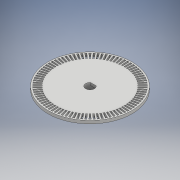
# Autodesk Inventor part: Ответная часть энкодера(колесо)
Saved by Autodesk Inventor 2018 (Build 220112000, 112)
## iProperties
Created: 2018-12-06
Part Number: Ответная часть энкодера(колесо)
Material: Типовые
Document SubType Name: Modeling
Designer: RR
Density: 1 g/cm^3
Appearance: По умолчанию
Author: RR
Autodesk Inventor part; units mm, degrees
ref_plane "YZ Plane" through (0, 0, 0) normal (1, 0, 0) x (0, 1, 0)
ref_plane "XZ Plane" through (0, 0, 0) normal (0, 1, 0) x (-1, 0, 0)
ref_plane "XY Plane" through (0, 0, 0) normal (0, 0, 1) x (1, 0, 0)
sketch "Эскиз1" plane through (0, 0, 0) normal (0, 0, 1) x (1, 0, 0)
  circle A0 centre (0, 0) radius 28
  arc A1 (1, 27.4818) -> (0, 27.5) centre (0, 0) ccw
  line L0 (0, 27.5) -> (1, 27.4818)
  arc A2 (0.8364, 22.9848) -> (0, 23) centre (0, 0) ccw
  line L1 (0, 2.3) -> (1.9261, 2.3) construction
  line L2 (1, 27.4818) -> (0.8364, 22.9848)
  line L3 (0, 23) -> (0, 27.5)
  arc A3 (-1.0087, 27.4815) -> (-2.0074, 27.4266) centre (0, 0) ccw
  line L4 (-2.0074, 27.4266) -> (-1.0087, 27.4815)
  arc A4 (-0.8436, 22.9845) -> (-1.6789, 22.9386) centre (0, 0) ccw
  line L5 (-1.0087, 27.4815) -> (-0.8436, 22.9845)
  line L6 (-1.6789, 22.9386) -> (-2.0074, 27.4266)
  arc A5 (-3.012, 27.3345) -> (-4.004, 27.2069) centre (0, 0) ccw
  line L7 (-4.004, 27.2069) -> (-3.012, 27.3345)
  arc A6 (-2.5192, 22.8616) -> (-3.3488, 22.7549) centre (0, 0) ccw
  line L8 (-3.012, 27.3345) -> (-2.5192, 22.8616)
  line L9 (-3.3488, 22.7549) -> (-4.004, 27.2069)
  arc A7 (-4.9993, 27.0418) -> (-5.9793, 26.8421) centre (0, 0) ccw
  line L10 (-5.9793, 26.8421) -> (-4.9993, 27.0418)
  arc A8 (-4.1812, 22.6167) -> (-5.0009, 22.4497) centre (0, 0) ccw
  line L11 (-4.9993, 27.0418) -> (-4.1812, 22.6167)
  line L12 (-5.0009, 22.4497) -> (-5.9793, 26.8421)
  arc A9 (-6.9599, 26.6047) -> (-7.9227, 26.334) centre (0, 0) ccw
  line L13 (-7.9227, 26.334) -> (-6.9599, 26.6047)
  arc A10 (-5.821, 22.2512) -> (-6.6263, 22.0248) centre (0, 0) ccw
  line L14 (-6.9599, 26.6047) -> (-5.821, 22.2512)
  line L15 (-6.6263, 22.0248) -> (-7.9227, 26.334)
  arc A11 (-8.8833, 26.0257) -> (-9.8238, 25.6854) centre (0, 0) ccw
  line L16 (-9.8238, 25.6854) -> (-8.8833, 26.0257)
  arc A12 (-7.4297, 21.7669) -> (-8.2163, 21.4824) centre (0, 0) ccw
  line L17 (-8.8833, 26.0257) -> (-7.4297, 21.7669)
  line L18 (-8.2163, 21.4824) -> (-9.8238, 25.6854)
  arc A13 (-10.7594, 25.3078) -> (-11.6726, 24.8998) centre (0, 0) ccw
  line L19 (-11.6726, 24.8998) -> (-10.7594, 25.3078)
  arc A14 (-8.9988, 21.1665) -> (-9.7625, 20.8253) centre (0, 0) ccw
  line L20 (-10.7594, 25.3078) -> (-8.9988, 21.1665)
  line L21 (-9.7625, 20.8253) -> (-11.6726, 24.8998)
  arc A15 (-12.578, 24.4549) -> (-13.459, 23.9814) centre (0, 0) ccw
  line L22 (-13.459, 23.9814) -> (-12.578, 24.4549)
  arc A16 (-10.5198, 20.4532) -> (-11.2566, 20.0571) centre (0, 0) ccw
  line L23 (-12.578, 24.4549) -> (-10.5198, 20.4532)
  line L24 (-11.2566, 20.0571) -> (-13.459, 23.9814)
  arc A17 (-14.3296, 23.4715) -> (-15.1736, 22.9349) centre (0, 0) ccw
  line L25 (-15.1736, 22.9349) -> (-14.3296, 23.4715)
  arc A18 (-11.9847, 19.6307) -> (-12.6907, 19.1819) centre (0, 0) ccw
  line L26 (-14.3296, 23.4715) -> (-11.9847, 19.6307)
  line L27 (-12.6907, 19.1819) -> (-15.1736, 22.9349)
  arc A19 (-16.0047, 22.3629) -> (-16.8073, 21.7662) centre (0, 0) ccw
  line L28 (-16.8073, 21.7662) -> (-16.0047, 22.3629)
  arc A20 (-13.3857, 18.7035) -> (-14.057, 18.2044) centre (0, 0) ccw
  line L29 (-16.0047, 22.3629) -> (-13.3857, 18.7035)
  line L30 (-14.057, 18.2044) -> (-16.8073, 21.7662)
  arc A21 (-17.5944, 21.135) -> (-18.3513, 20.4812) centre (0, 0) ccw
  line L31 (-18.3513, 20.4812) -> (-17.5944, 21.135)
  arc A22 (-14.7153, 17.6766) -> (-15.3483, 17.1298) centre (0, 0) ccw
  line L32 (-17.5944, 21.135) -> (-14.7153, 17.6766)
  line L33 (-15.3483, 17.1298) -> (-18.3513, 20.4812)
  arc A23 (-19.0902, 19.7943) -> (-19.7973, 19.087) centre (0, 0) ccw
  line L34 (-19.7973, 19.087) -> (-19.0902, 19.7943)
  arc A24 (-15.9663, 16.5552) -> (-16.5578, 15.9637) centre (0, 0) ccw
  line L35 (-19.0902, 19.7943) -> (-15.9663, 16.5552)
  line L36 (-16.5578, 15.9637) -> (-19.7973, 19.087)
  arc A25 (-20.4841, 18.348) -> (-21.1378, 17.591) centre (0, 0) ccw
  line L37 (-21.1378, 17.591) -> (-20.4841, 18.348)
  arc A26 (-17.1322, 15.3456) -> (-17.6789, 14.7125) centre (0, 0) ccw
  line L38 (-20.4841, 18.348) -> (-17.1322, 15.3456)
  line L39 (-17.6789, 14.7125) -> (-21.1378, 17.591)
  arc A27 (-21.7688, 16.8038) -> (-22.3655, 16.0011) centre (0, 0) ccw
  line L40 (-22.3655, 16.0011) -> (-21.7688, 16.8038)
  arc A28 (-18.2066, 14.0541) -> (-18.7057, 13.3828) centre (0, 0) ccw
  line L41 (-21.7688, 16.8038) -> (-18.2066, 14.0541)
  line L42 (-18.7057, 13.3828) -> (-22.3655, 16.0011)
  arc A29 (-22.9373, 15.17) -> (-23.4738, 14.3259) centre (0, 0) ccw
  line L43 (-23.4738, 14.3259) -> (-22.9373, 15.17)
  arc A30 (-19.184, 12.6876) -> (-19.6326, 11.9816) centre (0, 0) ccw
  line L44 (-22.9373, 15.17) -> (-19.184, 12.6876)
  line L45 (-19.6326, 11.9816) -> (-23.4738, 14.3259)
  arc A31 (-23.9835, 13.4552) -> (-24.4569, 12.5742) centre (0, 0) ccw
  line L46 (-24.4569, 12.5742) -> (-23.9835, 13.4552)
  arc A32 (-20.0589, 11.2534) -> (-20.4549, 10.5166) centre (0, 0) ccw
  line L47 (-23.9835, 13.4552) -> (-20.0589, 11.2534)
  line L48 (-20.4549, 10.5166) -> (-24.4569, 12.5742)
  arc A33 (-24.9017, 11.6686) -> (-25.3095, 10.7554) centre (0, 0) ccw
  line L49 (-25.3095, 10.7554) -> (-24.9017, 11.6686)
  arc A34 (-20.8269, 9.7592) -> (-21.168, 8.9954) centre (0, 0) ccw
  line L50 (-24.9017, 11.6686) -> (-20.8269, 9.7592)
  line L51 (-21.168, 8.9954) -> (-25.3095, 10.7554)
  arc A35 (-25.687, 9.8198) -> (-26.0271, 8.8792) centre (0, 0) ccw
  line L52 (-26.0271, 8.8792) -> (-25.687, 9.8198)
  arc A36 (-21.4837, 8.2129) -> (-21.7681, 7.4262) centre (0, 0) ccw
  line L53 (-25.687, 9.8198) -> (-21.4837, 8.2129)
  line L54 (-21.7681, 7.4262) -> (-26.0271, 8.8792)
  arc A37 (-26.3353, 7.9186) -> (-26.6058, 6.9557) centre (0, 0) ccw
  line L55 (-26.6058, 6.9557) -> (-26.3353, 7.9186)
  arc A38 (-22.0259, 6.6228) -> (-22.2521, 5.8175) centre (0, 0) ccw
  line L56 (-26.3353, 7.9186) -> (-22.0259, 6.6228)
  line L57 (-22.2521, 5.8175) -> (-26.6058, 6.9557)
  arc A39 (-26.843, 5.9751) -> (-27.0426, 4.995) centre (0, 0) ccw
  line L58 (-27.0426, 4.995) -> (-26.843, 5.9751)
  arc A40 (-22.4505, 4.9973) -> (-22.6174, 4.1776) centre (0, 0) ccw
  line L59 (-26.843, 5.9751) -> (-22.4505, 4.9973)
  line L60 (-22.6174, 4.1776) -> (-27.0426, 4.995)
  arc A41 (-27.2076, 3.9997) -> (-27.335, 3.0077) centre (0, 0) ccw
  line L61 (-27.335, 3.0077) -> (-27.2076, 3.9997)
  arc A42 (-22.7554, 3.3452) -> (-22.862, 2.5155) centre (0, 0) ccw
  line L62 (-27.2076, 3.9997) -> (-22.7554, 3.3452)
  line L63 (-22.862, 2.5155) -> (-27.335, 3.0077)
  arc A43 (-27.427, 2.003) -> (-27.4817, 1.0044) centre (0, 0) ccw
  line L64 (-27.4817, 1.0044) -> (-27.427, 2.003)
  arc A44 (-22.9389, 1.6753) -> (-22.9847, 0.84) centre (0, 0) ccw
  line L65 (-27.427, 2.003) -> (-22.9389, 1.6753)
  line L66 (-22.9847, 0.84) -> (-27.4817, 1.0044)
  arc A45 (-27.5, -0.0044) -> (-27.4817, -1.0044) centre (0, 0) ccw
  line L67 (-27.4817, -1.0044) -> (-27.5, -0.0044)
  arc A46 (-23, -0.0036) -> (-22.9847, -0.84) centre (0, 0) ccw
  line L68 (-27.5, -0.0044) -> (-23, -0.0036)
  line L69 (-22.9847, -0.84) -> (-27.4817, -1.0044)
  arc A47 (-27.4263, -2.0117) -> (-27.335, -3.0077) centre (0, 0) ccw
  line L70 (-27.335, -3.0077) -> (-27.4263, -2.0117)
  arc A48 (-22.9384, -1.6825) -> (-22.862, -2.5155) centre (0, 0) ccw
  line L71 (-27.4263, -2.0117) -> (-22.9384, -1.6825)
  line L72 (-22.862, -2.5155) -> (-27.335, -3.0077)
  arc A49 (-27.2063, -4.0083) -> (-27.0426, -4.995) centre (0, 0) ccw
  line L73 (-27.0426, -4.995) -> (-27.2063, -4.0083)
  arc A50 (-22.7544, -3.3524) -> (-22.6174, -4.1776) centre (0, 0) ccw
  line L74 (-27.2063, -4.0083) -> (-22.7544, -3.3524)
  line L75 (-22.6174, -4.1776) -> (-27.0426, -4.995)
  arc A51 (-26.8411, -5.9836) -> (-26.6058, -6.9557) centre (0, 0) ccw
  line L76 (-26.6058, -6.9557) -> (-26.8411, -5.9836)
  arc A52 (-22.449, -5.0045) -> (-22.2521, -5.8175) centre (0, 0) ccw
  line L77 (-26.8411, -5.9836) -> (-22.449, -5.0045)
  line L78 (-22.2521, -5.8175) -> (-26.6058, -6.9557)
  arc A53 (-26.3328, -7.9269) -> (-26.0271, -8.8792) centre (0, 0) ccw
  line L79 (-26.0271, -8.8792) -> (-26.3328, -7.9269)
  arc A54 (-22.0238, -6.6298) -> (-21.7681, -7.4262) centre (0, 0) ccw
  line L80 (-26.3328, -7.9269) -> (-22.0238, -6.6298)
  line L81 (-21.7681, -7.4262) -> (-26.0271, -8.8792)
  arc A55 (-25.6839, -9.8279) -> (-25.3095, -10.7554) centre (0, 0) ccw
  line L82 (-25.3095, -10.7554) -> (-25.6839, -9.8279)
  arc A56 (-21.4811, -8.2197) -> (-21.168, -8.9954) centre (0, 0) ccw
  line L83 (-25.6839, -9.8279) -> (-21.4811, -8.2197)
  line L84 (-21.168, -8.9954) -> (-25.3095, -10.7554)
  arc A57 (-24.898, -11.6765) -> (-24.4569, -12.5742) centre (0, 0) ccw
  line L85 (-24.4569, -12.5742) -> (-24.898, -11.6765)
  arc A58 (-20.8238, -9.7658) -> (-20.4549, -10.5166) centre (0, 0) ccw
  line L86 (-24.898, -11.6765) -> (-20.8238, -9.7658)
  line L87 (-20.4549, -10.5166) -> (-24.4569, -12.5742)
  arc A59 (-23.9792, -13.4628) -> (-23.4738, -14.3259) centre (0, 0) ccw
  line L88 (-23.4738, -14.3259) -> (-23.9792, -13.4628)
  arc A60 (-20.0554, -11.2598) -> (-19.6326, -11.9816) centre (0, 0) ccw
  line L89 (-23.9792, -13.4628) -> (-20.0554, -11.2598)
  line L90 (-19.6326, -11.9816) -> (-23.4738, -14.3259)
  arc A61 (-22.9325, -15.1772) -> (-22.3655, -16.0011) centre (0, 0) ccw
  line L91 (-22.3655, -16.0011) -> (-22.9325, -15.1772)
  arc A62 (-19.1799, -12.6937) -> (-18.7057, -13.3828) centre (0, 0) ccw
  line L92 (-22.9325, -15.1772) -> (-19.1799, -12.6937)
  line L93 (-18.7057, -13.3828) -> (-22.3655, -16.0011)
  arc A63 (-21.7635, -16.8107) -> (-21.1378, -17.591) centre (0, 0) ccw
  line L94 (-21.1378, -17.591) -> (-21.7635, -16.8107)
  arc A64 (-18.2022, -14.0599) -> (-17.6789, -14.7125) centre (0, 0) ccw
  line L95 (-21.7635, -16.8107) -> (-18.2022, -14.0599)
  line L96 (-17.6789, -14.7125) -> (-21.1378, -17.591)
  arc A65 (-20.4783, -18.3545) -> (-19.7973, -19.087) centre (0, 0) ccw
  line L97 (-19.7973, -19.087) -> (-20.4783, -18.3545)
  arc A66 (-17.1273, -15.351) -> (-16.5578, -15.9637) centre (0, 0) ccw
  line L98 (-20.4783, -18.3545) -> (-17.1273, -15.351)
  line L99 (-16.5578, -15.9637) -> (-19.7973, -19.087)
  arc A67 (-19.0839, -19.8004) -> (-18.3513, -20.4812) centre (0, 0) ccw
  line L100 (-18.3513, -20.4812) -> (-19.0839, -19.8004)
  arc A68 (-15.9611, -16.5603) -> (-15.3483, -17.1298) centre (0, 0) ccw
  line L101 (-19.0839, -19.8004) -> (-15.9611, -16.5603)
  line L102 (-15.3483, -17.1298) -> (-18.3513, -20.4812)
  arc A69 (-17.5877, -21.1406) -> (-16.8073, -21.7662) centre (0, 0) ccw
  line L103 (-16.8073, -21.7662) -> (-17.5877, -21.1406)
  arc A70 (-14.7097, -17.6812) -> (-14.057, -18.2044) centre (0, 0) ccw
  line L104 (-17.5877, -21.1406) -> (-14.7097, -17.6812)
  line L105 (-14.057, -18.2044) -> (-16.8073, -21.7662)
  arc A71 (-15.9976, -22.368) -> (-15.1736, -22.9349) centre (0, 0) ccw
  line L106 (-15.1736, -22.9349) -> (-15.9976, -22.368)
  arc A72 (-13.3798, -18.7078) -> (-12.6907, -19.1819) centre (0, 0) ccw
  line L107 (-15.9976, -22.368) -> (-13.3798, -18.7078)
  line L108 (-12.6907, -19.1819) -> (-15.1736, -22.9349)
  arc A73 (-14.3221, -23.4761) -> (-13.459, -23.9814) centre (0, 0) ccw
  line L109 (-13.459, -23.9814) -> (-14.3221, -23.4761)
  arc A74 (-11.9785, -19.6345) -> (-11.2566, -20.0571) centre (0, 0) ccw
  line L110 (-14.3221, -23.4761) -> (-11.9785, -19.6345)
  line L111 (-11.2566, -20.0571) -> (-13.459, -23.9814)
  arc A75 (-12.5703, -24.4589) -> (-11.6726, -24.8998) centre (0, 0) ccw
  line L112 (-11.6726, -24.8998) -> (-12.5703, -24.4589)
  arc A76 (-10.5133, -20.4565) -> (-9.7625, -20.8253) centre (0, 0) ccw
  line L113 (-12.5703, -24.4589) -> (-10.5133, -20.4565)
  line L114 (-9.7625, -20.8253) -> (-11.6726, -24.8998)
  arc A77 (-10.7514, -25.3112) -> (-9.8238, -25.6854) centre (0, 0) ccw
  line L115 (-9.8238, -25.6854) -> (-10.7514, -25.3112)
  arc A78 (-8.9921, -21.1694) -> (-8.2163, -21.4824) centre (0, 0) ccw
  line L116 (-10.7514, -25.3112) -> (-8.9921, -21.1694)
  line L117 (-8.2163, -21.4824) -> (-9.8238, -25.6854)
  arc A79 (-8.8751, -26.0285) -> (-7.9227, -26.334) centre (0, 0) ccw
  line L118 (-7.9227, -26.334) -> (-8.8751, -26.0285)
  arc A80 (-7.4228, -21.7693) -> (-6.6263, -22.0248) centre (0, 0) ccw
  line L119 (-8.8751, -26.0285) -> (-7.4228, -21.7693)
  line L120 (-6.6263, -22.0248) -> (-7.9227, -26.334)
  arc A81 (-6.9515, -26.6069) -> (-5.9793, -26.8421) centre (0, 0) ccw
  line L121 (-5.9793, -26.8421) -> (-6.9515, -26.6069)
  arc A82 (-5.8139, -22.253) -> (-5.0009, -22.4497) centre (0, 0) ccw
  line L122 (-6.9515, -26.6069) -> (-5.8139, -22.253)
  line L123 (-5.0009, -22.4497) -> (-5.9793, -26.8421)
  arc A83 (-4.9907, -27.0433) -> (-4.004, -27.2069) centre (0, 0) ccw
  line L124 (-4.004, -27.2069) -> (-4.9907, -27.0433)
  arc A84 (-4.1741, -22.6181) -> (-3.3488, -22.7549) centre (0, 0) ccw
  line L125 (-4.9907, -27.0433) -> (-4.1741, -22.6181)
  line L126 (-3.3488, -22.7549) -> (-4.004, -27.2069)
  arc A85 (-3.0034, -27.3355) -> (-2.0074, -27.4266) centre (0, 0) ccw
  line L127 (-2.0074, -27.4266) -> (-3.0034, -27.3355)
  arc A86 (-2.5119, -22.8624) -> (-1.6789, -22.9386) centre (0, 0) ccw
  line L128 (-3.0034, -27.3355) -> (-2.5119, -22.8624)
  line L129 (-1.6789, -22.9386) -> (-2.0074, -27.4266)
  arc A87 (-1, -27.4818) -> (0, -27.5) centre (0, 0) ccw
  line L130 (0, -27.5) -> (-1, -27.4818)
  arc A88 (-0.8364, -22.9848) -> (0, -23) centre (0, 0) ccw
  line L131 (-1, -27.4818) -> (-0.8364, -22.9848)
  line L132 (0, -23) -> (0, -27.5)
  arc A89 (1.0087, -27.4815) -> (2.0074, -27.4266) centre (0, 0) ccw
  line L133 (2.0074, -27.4266) -> (1.0087, -27.4815)
  arc A90 (0.8436, -22.9845) -> (1.6789, -22.9386) centre (0, 0) ccw
  line L134 (1.0087, -27.4815) -> (0.8436, -22.9845)
  line L135 (1.6789, -22.9386) -> (2.0074, -27.4266)
  arc A91 (3.012, -27.3345) -> (4.004, -27.2069) centre (0, 0) ccw
  line L136 (4.004, -27.2069) -> (3.012, -27.3345)
  arc A92 (2.5192, -22.8616) -> (3.3488, -22.7549) centre (0, 0) ccw
  line L137 (3.012, -27.3345) -> (2.5192, -22.8616)
  line L138 (3.3488, -22.7549) -> (4.004, -27.2069)
  arc A93 (4.9993, -27.0418) -> (5.9793, -26.8421) centre (0, 0) ccw
  line L139 (5.9793, -26.8421) -> (4.9993, -27.0418)
  arc A94 (4.1812, -22.6167) -> (5.0009, -22.4497) centre (0, 0) ccw
  line L140 (4.9993, -27.0418) -> (4.1812, -22.6167)
  line L141 (5.0009, -22.4497) -> (5.9793, -26.8421)
  arc A95 (6.9599, -26.6047) -> (7.9227, -26.334) centre (0, 0) ccw
  line L142 (7.9227, -26.334) -> (6.9599, -26.6047)
  arc A96 (5.821, -22.2512) -> (6.6263, -22.0248) centre (0, 0) ccw
  line L143 (6.9599, -26.6047) -> (5.821, -22.2512)
  line L144 (6.6263, -22.0248) -> (7.9227, -26.334)
  arc A97 (8.8833, -26.0257) -> (9.8238, -25.6854) centre (0, 0) ccw
  line L145 (9.8238, -25.6854) -> (8.8833, -26.0257)
  arc A98 (7.4297, -21.7669) -> (8.2163, -21.4824) centre (0, 0) ccw
  line L146 (8.8833, -26.0257) -> (7.4297, -21.7669)
  line L147 (8.2163, -21.4824) -> (9.8238, -25.6854)
  arc A99 (10.7594, -25.3078) -> (11.6726, -24.8998) centre (0, 0) ccw
  line L148 (11.6726, -24.8998) -> (10.7594, -25.3078)
  arc A100 (8.9988, -21.1665) -> (9.7625, -20.8253) centre (0, 0) ccw
  line L149 (10.7594, -25.3078) -> (8.9988, -21.1665)
  line L150 (9.7625, -20.8253) -> (11.6726, -24.8998)
  arc A101 (12.578, -24.4549) -> (13.459, -23.9814) centre (0, 0) ccw
  line L151 (13.459, -23.9814) -> (12.578, -24.4549)
  arc A102 (10.5198, -20.4532) -> (11.2566, -20.0571) centre (0, 0) ccw
  line L152 (12.578, -24.4549) -> (10.5198, -20.4532)
  line L153 (11.2566, -20.0571) -> (13.459, -23.9814)
  arc A103 (14.3296, -23.4715) -> (15.1736, -22.9349) centre (0, 0) ccw
  line L154 (15.1736, -22.9349) -> (14.3296, -23.4715)
  arc A104 (11.9847, -19.6307) -> (12.6907, -19.1819) centre (0, 0) ccw
  line L155 (14.3296, -23.4715) -> (11.9847, -19.6307)
  line L156 (12.6907, -19.1819) -> (15.1736, -22.9349)
  arc A105 (16.0047, -22.3629) -> (16.8073, -21.7662) centre (0, 0) ccw
  line L157 (16.8073, -21.7662) -> (16.0047, -22.3629)
  arc A106 (13.3857, -18.7035) -> (14.057, -18.2044) centre (0, 0) ccw
  line L158 (16.0047, -22.3629) -> (13.3857, -18.7035)
  line L159 (14.057, -18.2044) -> (16.8073, -21.7662)
  arc A107 (17.5944, -21.135) -> (18.3513, -20.4812) centre (0, 0) ccw
  line L160 (18.3513, -20.4812) -> (17.5944, -21.135)
  arc A108 (14.7153, -17.6766) -> (15.3483, -17.1298) centre (0, 0) ccw
  line L161 (17.5944, -21.135) -> (14.7153, -17.6766)
  line L162 (15.3483, -17.1298) -> (18.3513, -20.4812)
  arc A109 (19.0902, -19.7943) -> (19.7973, -19.087) centre (0, 0) ccw
  line L163 (19.7973, -19.087) -> (19.0902, -19.7943)
  arc A110 (15.9663, -16.5552) -> (16.5578, -15.9637) centre (0, 0) ccw
  line L164 (19.0902, -19.7943) -> (15.9663, -16.5552)
  line L165 (16.5578, -15.9637) -> (19.7973, -19.087)
  arc A111 (20.4841, -18.348) -> (21.1378, -17.591) centre (0, 0) ccw
  line L166 (21.1378, -17.591) -> (20.4841, -18.348)
  arc A112 (17.1322, -15.3456) -> (17.6789, -14.7125) centre (0, 0) ccw
  line L167 (20.4841, -18.348) -> (17.1322, -15.3456)
  line L168 (17.6789, -14.7125) -> (21.1378, -17.591)
  arc A113 (21.7688, -16.8038) -> (22.3655, -16.0011) centre (0, 0) ccw
  line L169 (22.3655, -16.0011) -> (21.7688, -16.8038)
  arc A114 (18.2066, -14.0541) -> (18.7057, -13.3828) centre (0, 0) ccw
  line L170 (21.7688, -16.8038) -> (18.2066, -14.0541)
  line L171 (18.7057, -13.3828) -> (22.3655, -16.0011)
  arc A115 (22.9373, -15.17) -> (23.4738, -14.3259) centre (0, 0) ccw
  line L172 (23.4738, -14.3259) -> (22.9373, -15.17)
  arc A116 (19.184, -12.6876) -> (19.6326, -11.9816) centre (0, 0) ccw
  line L173 (22.9373, -15.17) -> (19.184, -12.6876)
  line L174 (19.6326, -11.9816) -> (23.4738, -14.3259)
  arc A117 (23.9835, -13.4552) -> (24.4569, -12.5742) centre (0, 0) ccw
  line L175 (24.4569, -12.5742) -> (23.9835, -13.4552)
  arc A118 (20.0589, -11.2534) -> (20.4549, -10.5166) centre (0, 0) ccw
  line L176 (23.9835, -13.4552) -> (20.0589, -11.2534)
  line L177 (20.4549, -10.5166) -> (24.4569, -12.5742)
  arc A119 (24.9017, -11.6686) -> (25.3095, -10.7554) centre (0, 0) ccw
  line L178 (25.3095, -10.7554) -> (24.9017, -11.6686)
  arc A120 (20.8269, -9.7592) -> (21.168, -8.9954) centre (0, 0) ccw
  line L179 (24.9017, -11.6686) -> (20.8269, -9.7592)
  line L180 (21.168, -8.9954) -> (25.3095, -10.7554)
  arc A121 (25.687, -9.8198) -> (26.0271, -8.8792) centre (0, 0) ccw
  line L181 (26.0271, -8.8792) -> (25.687, -9.8198)
  arc A122 (21.4837, -8.2129) -> (21.7681, -7.4262) centre (0, 0) ccw
  line L182 (25.687, -9.8198) -> (21.4837, -8.2129)
  line L183 (21.7681, -7.4262) -> (26.0271, -8.8792)
  arc A123 (26.3353, -7.9186) -> (26.6058, -6.9557) centre (0, 0) ccw
  line L184 (26.6058, -6.9557) -> (26.3353, -7.9186)
  arc A124 (22.0259, -6.6228) -> (22.2521, -5.8175) centre (0, 0) ccw
  line L185 (26.3353, -7.9186) -> (22.0259, -6.6228)
  line L186 (22.2521, -5.8175) -> (26.6058, -6.9557)
  arc A125 (26.843, -5.9751) -> (27.0426, -4.995) centre (0, 0) ccw
  line L187 (27.0426, -4.995) -> (26.843, -5.9751)
  arc A126 (22.4505, -4.9973) -> (22.6174, -4.1776) centre (0, 0) ccw
  line L188 (26.843, -5.9751) -> (22.4505, -4.9973)
  line L189 (22.6174, -4.1776) -> (27.0426, -4.995)
  arc A127 (27.2076, -3.9997) -> (27.335, -3.0077) centre (0, 0) ccw
  line L190 (27.335, -3.0077) -> (27.2076, -3.9997)
  arc A128 (22.7554, -3.3452) -> (22.862, -2.5155) centre (0, 0) ccw
  line L191 (27.2076, -3.9997) -> (22.7554, -3.3452)
  line L192 (22.862, -2.5155) -> (27.335, -3.0077)
  arc A129 (27.427, -2.003) -> (27.4817, -1.0044) centre (0, 0) ccw
  line L193 (27.4817, -1.0044) -> (27.427, -2.003)
  arc A130 (22.9389, -1.6753) -> (22.9847, -0.84) centre (0, 0) ccw
  line L194 (27.427, -2.003) -> (22.9389, -1.6753)
  line L195 (22.9847, -0.84) -> (27.4817, -1.0044)
  arc A131 (27.5, 0.0044) -> (27.4817, 1.0044) centre (0, 0) ccw
  line L196 (27.4817, 1.0044) -> (27.5, 0.0044)
  arc A132 (23, 0.0036) -> (22.9847, 0.84) centre (0, 0) ccw
  line L197 (27.5, 0.0044) -> (23, 0.0036)
  line L198 (22.9847, 0.84) -> (27.4817, 1.0044)
  arc A133 (27.4263, 2.0117) -> (27.335, 3.0077) centre (0, 0) ccw
  line L199 (27.335, 3.0077) -> (27.4263, 2.0117)
  arc A134 (22.9384, 1.6825) -> (22.862, 2.5155) centre (0, 0) ccw
  line L200 (27.4263, 2.0117) -> (22.9384, 1.6825)
  line L201 (22.862, 2.5155) -> (27.335, 3.0077)
  arc A135 (27.2063, 4.0083) -> (27.0426, 4.995) centre (0, 0) ccw
  line L202 (27.0426, 4.995) -> (27.2063, 4.0083)
  arc A136 (22.7544, 3.3524) -> (22.6174, 4.1776) centre (0, 0) ccw
  line L203 (27.2063, 4.0083) -> (22.7544, 3.3524)
  line L204 (22.6174, 4.1776) -> (27.0426, 4.995)
  arc A137 (26.8411, 5.9836) -> (26.6058, 6.9557) centre (0, 0) ccw
  line L205 (26.6058, 6.9557) -> (26.8411, 5.9836)
  arc A138 (22.449, 5.0045) -> (22.2521, 5.8175) centre (0, 0) ccw
  line L206 (26.8411, 5.9836) -> (22.449, 5.0045)
  line L207 (22.2521, 5.8175) -> (26.6058, 6.9557)
  arc A139 (26.3328, 7.9269) -> (26.0271, 8.8792) centre (0, 0) ccw
  line L208 (26.0271, 8.8792) -> (26.3328, 7.9269)
  arc A140 (22.0238, 6.6298) -> (21.7681, 7.4262) centre (0, 0) ccw
  line L209 (26.3328, 7.9269) -> (22.0238, 6.6298)
  line L210 (21.7681, 7.4262) -> (26.0271, 8.8792)
  arc A141 (25.6839, 9.8279) -> (25.3095, 10.7554) centre (0, 0) ccw
  line L211 (25.3095, 10.7554) -> (25.6839, 9.8279)
  arc A142 (21.4811, 8.2197) -> (21.168, 8.9954) centre (0, 0) ccw
  line L212 (25.6839, 9.8279) -> (21.4811, 8.2197)
  line L213 (21.168, 8.9954) -> (25.3095, 10.7554)
  arc A143 (24.898, 11.6765) -> (24.4569, 12.5742) centre (0, 0) ccw
  line L214 (24.4569, 12.5742) -> (24.898, 11.6765)
  arc A144 (20.8238, 9.7658) -> (20.4549, 10.5166) centre (0, 0) ccw
  line L215 (24.898, 11.6765) -> (20.8238, 9.7658)
  line L216 (20.4549, 10.5166) -> (24.4569, 12.5742)
  arc A145 (23.9792, 13.4628) -> (23.4738, 14.3259) centre (0, 0) ccw
  line L217 (23.4738, 14.3259) -> (23.9792, 13.4628)
  arc A146 (20.0554, 11.2598) -> (19.6326, 11.9816) centre (0, 0) ccw
  line L218 (23.9792, 13.4628) -> (20.0554, 11.2598)
  line L219 (19.6326, 11.9816) -> (23.4738, 14.3259)
  arc A147 (22.9325, 15.1772) -> (22.3655, 16.0011) centre (0, 0) ccw
  line L220 (22.3655, 16.0011) -> (22.9325, 15.1772)
  arc A148 (19.1799, 12.6937) -> (18.7057, 13.3828) centre (0, 0) ccw
  line L221 (22.9325, 15.1772) -> (19.1799, 12.6937)
  line L222 (18.7057, 13.3828) -> (22.3655, 16.0011)
  arc A149 (21.7635, 16.8107) -> (21.1378, 17.591) centre (0, 0) ccw
  line L223 (21.1378, 17.591) -> (21.7635, 16.8107)
  arc A150 (18.2022, 14.0599) -> (17.6789, 14.7125) centre (0, 0) ccw
  line L224 (21.7635, 16.8107) -> (18.2022, 14.0599)
  line L225 (17.6789, 14.7125) -> (21.1378, 17.591)
  arc A151 (20.4783, 18.3545) -> (19.7973, 19.087) centre (0, 0) ccw
  line L226 (19.7973, 19.087) -> (20.4783, 18.3545)
  arc A152 (17.1273, 15.351) -> (16.5578, 15.9637) centre (0, 0) ccw
  line L227 (20.4783, 18.3545) -> (17.1273, 15.351)
  line L228 (16.5578, 15.9637) -> (19.7973, 19.087)
  arc A153 (19.0839, 19.8004) -> (18.3513, 20.4812) centre (0, 0) ccw
  line L229 (18.3513, 20.4812) -> (19.0839, 19.8004)
  arc A154 (15.9611, 16.5603) -> (15.3483, 17.1298) centre (0, 0) ccw
  line L230 (19.0839, 19.8004) -> (15.9611, 16.5603)
  line L231 (15.3483, 17.1298) -> (18.3513, 20.4812)
  arc A155 (17.5877, 21.1406) -> (16.8073, 21.7662) centre (0, 0) ccw
  line L232 (16.8073, 21.7662) -> (17.5877, 21.1406)
  arc A156 (14.7097, 17.6812) -> (14.057, 18.2044) centre (0, 0) ccw
  line L233 (17.5877, 21.1406) -> (14.7097, 17.6812)
  line L234 (14.057, 18.2044) -> (16.8073, 21.7662)
  arc A157 (15.9976, 22.368) -> (15.1736, 22.9349) centre (0, 0) ccw
  line L235 (15.1736, 22.9349) -> (15.9976, 22.368)
  arc A158 (13.3798, 18.7078) -> (12.6907, 19.1819) centre (0, 0) ccw
  line L236 (15.9976, 22.368) -> (13.3798, 18.7078)
  line L237 (12.6907, 19.1819) -> (15.1736, 22.9349)
  arc A159 (14.3221, 23.4761) -> (13.459, 23.9814) centre (0, 0) ccw
  line L238 (13.459, 23.9814) -> (14.3221, 23.4761)
  arc A160 (11.9785, 19.6345) -> (11.2566, 20.0571) centre (0, 0) ccw
  line L239 (14.3221, 23.4761) -> (11.9785, 19.6345)
  line L240 (11.2566, 20.0571) -> (13.459, 23.9814)
  arc A161 (12.5703, 24.4589) -> (11.6726, 24.8998) centre (0, 0) ccw
  line L241 (11.6726, 24.8998) -> (12.5703, 24.4589)
  arc A162 (10.5133, 20.4565) -> (9.7625, 20.8253) centre (0, 0) ccw
  line L242 (12.5703, 24.4589) -> (10.5133, 20.4565)
  line L243 (9.7625, 20.8253) -> (11.6726, 24.8998)
  arc A163 (10.7514, 25.3112) -> (9.8238, 25.6854) centre (0, 0) ccw
  line L244 (9.8238, 25.6854) -> (10.7514, 25.3112)
  arc A164 (8.9921, 21.1694) -> (8.2163, 21.4824) centre (0, 0) ccw
  line L245 (10.7514, 25.3112) -> (8.9921, 21.1694)
  line L246 (8.2163, 21.4824) -> (9.8238, 25.6854)
  arc A165 (8.8751, 26.0285) -> (7.9227, 26.334) centre (0, 0) ccw
  line L247 (7.9227, 26.334) -> (8.8751, 26.0285)
  arc A166 (7.4228, 21.7693) -> (6.6263, 22.0248) centre (0, 0) ccw
  line L248 (8.8751, 26.0285) -> (7.4228, 21.7693)
  line L249 (6.6263, 22.0248) -> (7.9227, 26.334)
  arc A167 (6.9515, 26.6069) -> (5.9793, 26.8421) centre (0, 0) ccw
  line L250 (5.9793, 26.8421) -> (6.9515, 26.6069)
  arc A168 (5.8139, 22.253) -> (5.0009, 22.4497) centre (0, 0) ccw
  line L251 (6.9515, 26.6069) -> (5.8139, 22.253)
  line L252 (5.0009, 22.4497) -> (5.9793, 26.8421)
  arc A169 (4.9907, 27.0433) -> (4.004, 27.2069) centre (0, 0) ccw
  line L253 (4.004, 27.2069) -> (4.9907, 27.0433)
  arc A170 (4.1741, 22.6181) -> (3.3488, 22.7549) centre (0, 0) ccw
  line L254 (4.9907, 27.0433) -> (4.1741, 22.6181)
  line L255 (3.3488, 22.7549) -> (4.004, 27.2069)
  arc A171 (3.0034, 27.3355) -> (2.0074, 27.4266) centre (0, 0) ccw
  line L256 (2.0074, 27.4266) -> (3.0034, 27.3355)
  arc A172 (2.5119, 22.8624) -> (1.6789, 22.9386) centre (0, 0) ccw
  line L257 (3.0034, 27.3355) -> (2.5119, 22.8624)
  line L258 (1.6789, 22.9386) -> (2.0074, 27.4266)
  line L259 (-1.9261, 2.3) -> (1.9261, 2.3)
  arc A173 (-1.9261, 2.3) -> (1.9261, 2.3) centre (0, 0) ccw
  line L260 (-1.9261, 2.3) -> (1.9261, 2.3)
  dimension "d9" = 360
  dimension "d11" = 6
  constraints: 522 end point, 346 point on circle, 174 centre point, 88 coincident, 2 horizontal, 1 collinear, 1 vertical, 947 other
  measures "d11" diameter of A173
extrude "Выдавливание1" add sketch "Эскиз1" along normal blind 2
sketch "Эскиз2" plane through (0, 0, 0) normal (0, 0, -1) x (-1, 0, 0)
  circle A0 centre (0, 0) radius 3
  constraints: 1 centre point, 1 coincident
extrude "Выдавливание2" cut sketch "Эскиз2" against normal blind 1
sketch "Эскиз3" plane through (0, 0, 0) normal (0, 0, -1) x (-1, 0, 0)
  circle A0 centre (0, 0) radius 3 projected
  circle A1 centre (0, 0) radius 28
  circle A2 centre (0, 0) radius 28.5
  dimension "d16" = 57
  constraints: 2 centre point, 2 coincident
  measures "d16" diameter of A2
extrude "Выдавливание3" add sketch "Эскиз3" against normal blind 2 contours A2
sketch "Эскиз4" plane through (0, 0, 0) normal (0, 0, -1) x (-1, 0, 0)
  circle A0 centre (0, 0) radius 3
  circle A1 centre (0, 0) radius 7
  constraints: 2 centre point, 2 coincident
sketch "Эскиз5" plane through (-9.8238, 25.6854, 2) normal (0.9340161, 0.3572309, 0) x (0, 0, -1)
  line L0 (2, -4.5152) -> (2, -4.5) projected
  line L1 (2, -24.5) -> (4, -24.5)
  line L2 (4, -24.5) -> (2, -7)
  line L3 (2, -24.5) -> (2, -7)
  line L4 (2, -27.5) -> (6, -27.5)
  dimension "d19" = 2
  constraints: 8 end point, 2 horizontal, 1 vertical
  measures "d19" distance of L1.start L1.end
revolve "Вращение1" add sketch "Эскиз5" angle 360 about axis through (0, 0, 0) along (0, 0, -1)
extrude "Выдавливание4" add sketch "Эскиз4" along normal blind 2.5
sketch "Эскиз6" plane through (0, 0, 1) normal (0, 0, -1) x (-1, 0, 0)
  arc A0 (1.9261, 2.3) -> (-1.9261, 2.3) centre (0, 0) ccw projected
  line L0 (1.9261, 2.3) -> (-1.9261, 2.3) projected
  line L1 (1.9261, 2.3) -> (1.9261, 2.3)
  arc A1 (1.9261, 2.3) -> (-1.9261, 2.3) centre (0, 0) ccw
  constraints: 2 end point, 2 point on circle, 1 centre point, 1 collinear, 1 concentric
extrude "Выдавливание5" add sketch "Эскиз6" along normal blind 0.8
chamfer "Фаска1" distance 0.95 angle 45 1 edges at (7, 0, -2.5)
